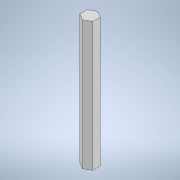
# Autodesk Inventor part: Part8
Saved by Autodesk Inventor 2022 (Build 260153000, 153)
## iProperties
Created: 2022-12-05
Part Number: Part8
Material: Generic
Document SubType Name: Modeling
Designer: s135320
Density: 1 g/cm^3
Appearance: Default
Author: s135320
Autodesk Inventor part; units mm, degrees
ref_plane "YZ Plane" through (0, 0, 0) normal (1, 0, 0) x (0, 1, 0)
ref_plane "XZ Plane" through (0, 0, 0) normal (0, 1, 0) x (-1, 0, 0)
ref_plane "XY Plane" through (0, 0, 0) normal (0, 0, 1) x (1, 0, 0)
sketch "Sketch1" plane through (0, 0, 0) normal (0, 1, 0) x (-1, 0, 0)
  line L0 (0, -7.3152) -> (-6.3351, -3.6576)
  line L1 (-6.3351, -3.6576) -> (-6.3351, 3.6576)
  line L2 (-6.3351, 3.6576) -> (0, 7.3152)
  line L3 (0, 7.3152) -> (6.3351, 3.6576)
  line L4 (6.3351, 3.6576) -> (6.3351, -3.6576)
  line L5 (6.3351, -3.6576) -> (0, -7.3152)
  point P0 (0, 0)
  point P1 (0, 0)
  dimension "d0" = 7.3152
  constraints: 12 end point, 1 coincident, 13 other
  measures "d0" distance of L3.end L4.end
extrude "Extrusion1" add sketch "Sketch1" along normal blind 127
body "Solid1"
